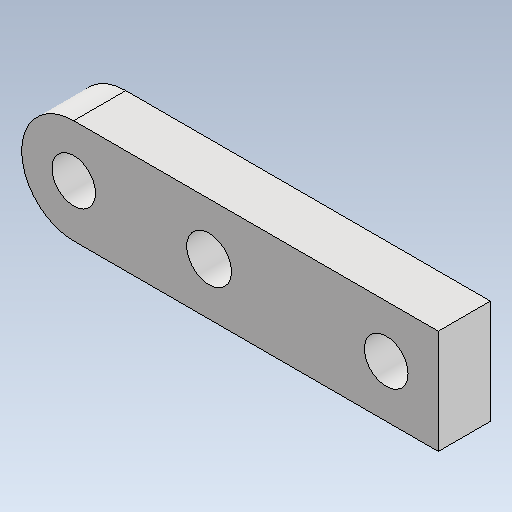
# Autodesk Inventor part: gate-pivot
Saved by Autodesk Inventor 2025 (Build 290162000, 162)
## iProperties
Created: 2025-08-22
Part Number: gate-pivot
Material: Generic
Document SubType Name: Modeling
Designer: HP
Density: 1 g/cm^3
Appearance: Default
Author: HP
Autodesk Inventor part; units mm, degrees
ref_plane "YZ Plane" through (0, 0, 0) normal (1, 0, 0) x (0, 1, 0)
ref_plane "XZ Plane" through (0, 0, 0) normal (0, 1, 0) x (-1, 0, 0)
ref_plane "XY Plane" through (0, 0, 0) normal (0, 0, 1) x (1, 0, 0)
sketch "Sketch1" plane through (0, 0, 0) normal (0, 0, 1) x (1, 0, 0)
  line L0 (-15, 0) -> (15, 0) construction
  line L1 (-15, -5) -> (20, -5)
  line L2 (20, 5) -> (-15, 5)
  arc A0 (-15, 5) -> (-15, -5) centre (-15, 0) ccw
  arc A1 (15, -5) -> (15, 5) centre (15, 0) ccw construction
  circle A2 centre (-15, 0) radius 2.1
  circle A3 centre (15, 0) radius 2.1
  circle A4 centre (-2, 0) radius 2.15
  line L3 (20, 5) -> (20, -5)
  point P0 (0, 0)
  point P1 (0, 0)
  dimension "d0" = 5
  dimension "d1" = 4.2
  dimension "d2" = 4.2
  dimension "d3" = 30
  dimension "d6" = 4.3
  dimension "d7" = 17
  constraints: 10 end point, 5 centre point, 5 tangent, 4 point on circle, 3 coincident, 3 point on line, 1 horizontal, 1 midpoint, 1 parallel, 1 vertical
  measures "d0" radius of A1
  measures "d1" diameter of A2
  measures "d2" diameter of A3
  measures "d3" distance of L0.start L0.end
  measures "d6" diameter of A4
  measures "d7" distance of L0.end A4.centre
extrude "Extrusion1" add sketch "Sketch1" along normal blind 5
body "Solid1"
